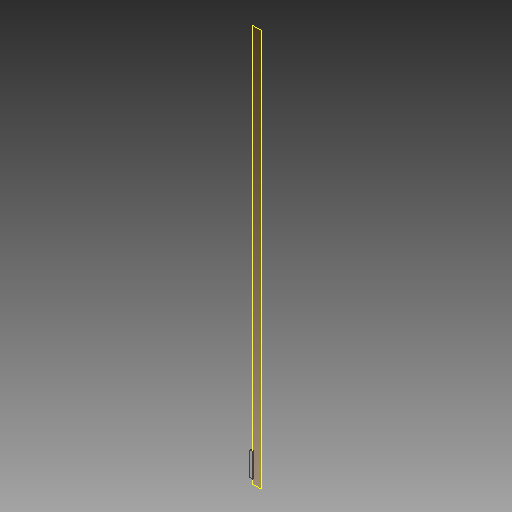
# Autodesk Inventor part: afstandsstykke
Saved by Autodesk Inventor 2018 (Build 220112000, 112)
## iProperties
Created: 2019-09-28
Part Number: afstandsstykke
Material: S235JR
Document SubType Name: Modeling
Designer: loppen
Density: 7.85 g/cm^3
Appearance: Light Gray
Mass: 25.12 g
Surface Area: 23.2 cm^2
Volume: 3.2 cm^3
Author: loppen
Autodesk Inventor part; units mm, degrees
ref_plane "YZ Plane" through (0, 0, 0) normal (1, 0, 0) x (0, 1, 0)
ref_plane "XZ Plane" through (0, 0, 0) normal (0, 1, 0) x (-1, 0, 0)
ref_plane "XY Plane" through (0, 0, 0) normal (0, 0, 1) x (1, 0, 0)
ref_plane "Work Plane1" through (0, 0, 0) normal (0, 0, 1) x (1, 0, 0)
sketch "Sketch1" plane through (0, 0, 0) normal (0, 0, 1) x (1, 0, 0)
  line L0 (-11.1078, -570.4657) -> (-1.1078, -570.4657)
  line L1 (-1.1078, -570.4657) -> (-1.1078, -650.4657)
  line L2 (-1.1078, -650.4657) -> (-11.1078, -650.4657)
  line L3 (-11.1078, -650.4657) -> (-11.1078, -570.4657)
  point P0 (0, 0)
  dimension "d0" = 10
  dimension "d1" = 80
  constraints: 8 end point, 2 horizontal, 2 parallel, 1 perpendicular, 1 vertical
  measures "d0" distance of L0.start L0.end
  measures "d1" distance of L0.end L1.end
extrude "Extrusion1" add sketch "Sketch1" against normal blind 4
body "Solid1"
